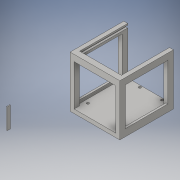
# Autodesk Inventor part: Frame_+_Slide_Top
Saved by Autodesk Inventor 2016 (Build 200138000, 138)
## iProperties
Created: 2018-09-16
Part Number: Frame_+_Slide_Top
Material: Generic
Document SubType Name: Modeling
Designer: Kyle
Density: 1 g/cm^3
Appearance: Default
Author: Kyle
Autodesk Inventor part; units mm, degrees
ref_plane "YZ Plane" through (0, 0, 0) normal (1, 0, 0) x (0, 1, 0)
ref_plane "XZ Plane" through (0, 0, 0) normal (0, 1, 0) x (-1, 0, 0)
ref_plane "XY Plane" through (0, 0, 0) normal (0, 0, 1) x (1, 0, 0)
sketch "Sketch1" plane through (0, 0, 0) normal (0, 1, 0) x (-1, 0, 0)
  line L0 (-26.5, 34) -> (26.5, 34)
  line L1 (26.5, 34) -> (26.5, -34)
  line L2 (26.5, -34) -> (-26.5, -34)
  line L3 (-26.5, -34) -> (-26.5, 34)
  line L4 (-26.5, 34) -> (26.5, -34) construction
  line L5 (26.5, 34) -> (-26.5, -34) construction
  line L6 (26.5, 34) -> (26.5, 19)
  line L7 (-26.5, -34) -> (-19.5, -34)
  line L8 (-26.5, -34) -> (8.5, -34)
  circle A0 centre (8.5, -31.5) radius 1.5
  circle A1 centre (-19.5, -31.5) radius 1.5
  line L9 (-19.5, -33) -> (-19.5, -34)
  line L10 (8.5, -33) -> (8.5, -34)
  circle A2 centre (-19.5, -31.5) radius 1.5
  circle A3 centre (24, 19) radius 1.5
  line L11 (25.5, 19) -> (26.5, 19)
  line L12 (26.5, 19) -> (25.5, 19)
  line L13 (24, 19) -> (0, 19)
  line L14 (0, 19) -> (0, 0)
  line L15 (0, 0) -> (8.5, -31.5)
  line L16 (8.5, -31.5) -> (0, -31.5)
  line L17 (-19.5, -31.5) -> (-19.5, 0)
  line L18 (-19.5, 0) -> (0, 0)
  line L19 (26.5, 34) -> (31.5, 34)
  line L20 (-31.5, -34) -> (31.5, -34)
  line L21 (31.5, -34) -> (31.5, 34)
  line L22 (31.5, 34) -> (-31.5, 34)
  line L23 (-31.5, 34) -> (-31.5, -34)
  line L24 (-31.5, -34) -> (31.5, 34) construction
  line L25 (31.5, -34) -> (-31.5, 34) construction
  dimension "d5" = 3
  dimension "d6" = 3
  dimension "d7" = 3
  dimension "d0" = 53
  dimension "d1" = 68
  dimension "d2" = 15
  dimension "d3" = 7
  dimension "d4" = 35
  dimension "d8" = 1
  dimension "d9" = 1
  dimension "d10" = 5
  constraints: 52 end point, 5 parallel, 5 perpendicular, 5 point on line, 4 midpoint, 3 horizontal, 2 vertical, 2 vertical alignment, 1 centre point, 1 coincident, 1 collinear, 1 horizontal alignment, 7 other
  measures "d0" distance of L1.end L2.end
  measures "d1" distance of L0.end L1.end
  measures "d2" distance of L0.end L6.end
  measures "d3" distance of L2.end L7.end
  measures "d4" distance of L2.end L8.end
  measures "d8" distance of L10.start L8.end
  measures "d9" distance of L11.start L6.end
  measures "d10" distance of L0.end L19.end
extrude "Extrusion1" add sketch "Sketch1" along normal blind 5 contours L0 L1 L11 A3 L13 L14 L18 L17 A1 L9 L2 L3 | L3 L20 L23 L22 | L19 L21 L20 L1 | L1 L2 L10 A0 L15 L14 L13 A3 L11 | L9 A1 L17 L18 L15 A0 L10 L2
sketch "Sketch2" plane through (0, 0, 0) normal (0, 1, 0) x (-1, 0, 0)
  line L0 (51.0115, 95.1402) -> (50.0115, 95.1402)
  line L1 (50.0115, 95.1402) -> (50.0115, 90.9953)
  line L2 (50.0115, 90.9953) -> (51.0115, 90.9953)
  line L3 (51.0115, 90.9953) -> (51.0115, 95.1402)
  point P0 (0, 0)
  dimension "d13" = 1
  constraints: 8 end point, 2 parallel, 1 horizontal, 1 perpendicular
  measures "d13" distance of L2.end L1.end
extrude "Extrusion2" add sketch "Sketch2" along normal blind 26
sketch "Sketch3" plane through (0, 5, 0) normal (0, 1, 0) x (1, 0, 0)
  line L0 (31.5, -34) -> (-31.5, -34)
  line L1 (-31.5, -34) -> (-31.5, 34)
  line L2 (-31.5, 34) -> (31.5, 34)
  line L3 (31.5, 34) -> (31.5, -34)
  line L4 (31.5, -34) -> (-31.5, 34) construction
  line L5 (-31.5, -34) -> (31.5, 34) construction
  line L6 (-31.5, -34) -> (31.5, -34) projected
  line L7 (-31.5, 34) -> (-26.5, 34)
  line L8 (-26.5, 34) -> (-26.5, -34)
  line L9 (-26.5, -34) -> (-31.5, -34)
  line L10 (-31.5, -34) -> (-31.5, 34)
  line L11 (31.5, -34) -> (31.5, 34) projected
  line L12 (31.5, 34) -> (26.5, 34)
  line L13 (26.5, 34) -> (26.5, -34)
  line L14 (26.5, -34) -> (31.5, -34)
  line L15 (31.5, -34) -> (31.5, 34)
  line L16 (-31.5, -34) -> (-26.5, -34)
  line L17 (-26.5, -34) -> (-26.5, -27)
  line L18 (-26.5, -27) -> (-31.5, -27)
  line L19 (-31.5, -27) -> (-31.5, -34)
  line L20 (-31.5, 34) -> (-26.5, 34)
  line L21 (-26.5, 34) -> (-26.5, 27)
  line L22 (-26.5, 27) -> (-31.5, 27)
  line L23 (-31.5, 27) -> (-31.5, 34)
  line L24 (31.5, 34) -> (26.5, 34)
  line L25 (26.5, 34) -> (26.5, 27)
  line L26 (26.5, 27) -> (31.5, 27)
  line L27 (31.5, 27) -> (31.5, 34)
  line L28 (26.5, -34) -> (31.5, -34)
  line L29 (31.5, -34) -> (31.5, -27)
  line L30 (31.5, -27) -> (26.5, -27)
  line L31 (26.5, -27) -> (26.5, -34)
  point P0 (0, 0)
  dimension "d16" = 5
  dimension "d17" = 5
  dimension "d18" = 5
  dimension "d19" = 7
  dimension "d20" = 5
  dimension "d21" = 7
  dimension "d22" = 5
  dimension "d23" = 7
  dimension "d24" = 5
  dimension "d25" = 7
  constraints: 60 end point, 14 parallel, 7 horizontal, 7 perpendicular, 2 midpoint, 2 point on line
  measures "d16" distance of L8.end L9.end
  measures "d17" distance of L14.end L13.end
  measures "d18" distance of L18.end L17.end
  measures "d19" distance of L17.end L16.end
  measures "d20" distance of L21.end L22.end
  measures "d21" distance of L20.end L21.end
  measures "d22" distance of L26.end L25.end
  measures "d23" distance of L25.end L24.end
  measures "d24" distance of L30.end L29.end
  measures "d25" distance of L29.end L28.end
extrude "Extrusion3" add sketch "Sketch3" along normal blind 52 contours L0 L13 L30 L3 | L0 L1 L18 L8 | L26 L13 L2 L3 | L22 L1 L2 L8
sketch "Sketch4" plane through (0, 5, 0) normal (0, 1, 0) x (1, 0, 0)
  line L0 (-31.5, 27) -> (-31.5, -27) projected
  line L1 (-26.5, -27) -> (-26.5, -34) projected
  line L2 (-31.5, 27) -> (-26.5, 27)
  line L3 (-26.5, 27) -> (-26.5, -27)
  line L4 (-26.5, -27) -> (-31.5, -27)
  line L5 (-31.5, -27) -> (-31.5, 27)
  line L6 (31.5, -27) -> (31.5, 27) projected
  line L7 (31.5, 27) -> (26.5, 27)
  line L8 (26.5, 27) -> (26.5, -27)
  line L9 (26.5, -27) -> (31.5, -27)
  line L10 (31.5, -27) -> (31.5, 27)
  line L11 (31.5, -27) -> (26.5, -27) projected
  line L12 (31.5, 27) -> (29, 27)
  line L13 (29, 27) -> (29, -27)
  line L14 (29, -27) -> (31.5, -27)
  line L15 (31.5, -27) -> (31.5, 27)
  line L16 (-26.5, -27) -> (-31.5, -27) projected
  line L17 (-31.5, 27) -> (-29, 27)
  line L18 (-29, 27) -> (-29, -27)
  line L19 (-29, -27) -> (-31.5, -27)
  line L20 (-31.5, -27) -> (-31.5, 27)
  point P0 (0, 0)
  constraints: 32 end point, 8 parallel, 4 horizontal, 4 perpendicular, 2 midpoint
extrude "Extrusion4" add sketch "Sketch4" along normal blind 4 contours L2 L18 L4 L0 | L9 L13 L7 L6
sketch "Sketch5" plane through (0, 57, 0) normal (0, 1, 0) x (1, 0, 0)
  line L0 (31.5, 34) -> (-31.5, 34) projected
  line L1 (-26.5, -34) -> (-26.5, -27) projected
  line L2 (-31.5, 34) -> (-26.5, 34)
  line L3 (-26.5, 34) -> (-26.5, -34)
  line L4 (-26.5, -34) -> (-31.5, -34)
  line L5 (-31.5, -34) -> (-31.5, 34)
  line L6 (-26.5, -27) -> (31.5, -27)
  line L7 (31.5, -27) -> (31.5, -34)
  line L8 (31.5, -34) -> (-26.5, -34)
  line L9 (-26.5, -34) -> (-26.5, -27)
  line L10 (26.5, -27) -> (26.5, -34) projected
  line L11 (26.5, -27) -> (31.5, -27)
  line L12 (31.5, -27) -> (31.5, 34)
  line L13 (31.5, 34) -> (26.5, 34)
  line L14 (26.5, 34) -> (26.5, -27)
  line L15 (-26.5, 27) -> (-26.5, 34) projected
  line L16 (-26.5, 34) -> (-26.5, 27)
  line L17 (26.5, 27) -> (26.5, 34)
  point P0 (0, 0)
  constraints: 28 end point, 7 parallel, 3 horizontal, 3 perpendicular, 1 point on line
extrude "Extrusion5" add sketch "Sketch5" along normal blind 8 contours L12 L6 L14 L0 | L7 L8 L10 L6 | L3 L1 L4 L5 L0 | L10 L8 L1 L6
sketch "Sketch6" plane through (31.5, 0, -34) normal (0, 0, -1) x (-1, 0, 0)
  line L0 (0, 0) -> (0, 65) projected
  line L1 (5, 5) -> (5, 57) projected
  line L2 (0, 65) -> (5, 65)
  line L3 (5, 63) -> (5, 60)
  line L4 (5, 57) -> (0, 57)
  line L5 (0, 57) -> (0, 65)
  line L6 (58, 5) -> (58, 57) projected
  line L7 (63, 0) -> (63, 65) projected
  line L8 (58, 57) -> (63, 57)
  line L9 (63, 57) -> (63, 65)
  line L10 (63, 65) -> (58, 65)
  line L11 (58, 65) -> (58, 57)
  line L12 (5, 57) -> (5, 60)
  line L13 (5, 5) -> (5, 65) projected
  line L14 (5, 60) -> (2.5, 60)
  line L15 (2.5, 60) -> (2.5, 63)
  line L16 (2.5, 63) -> (5, 63)
  line L17 (58, 57) -> (5, 57) projected
  line L18 (58, 57) -> (60.5, 57)
  line L19 (63, 57) -> (58, 57) projected
  line L20 (60.5, 60) -> (58, 60)
  line L21 (58, 5) -> (58, 65) projected
  line L22 (58, 60) -> (58, 63)
  line L23 (58, 63) -> (60.5, 63)
  line L24 (60.5, 63) -> (60.5, 60)
  line L25 (5, 63) -> (5, 60)
  point P0 (31.5, 0)
  point P1 (59.25, 63)
  point P2 (59.25, 60)
  dimension "d32" = 3
  dimension "d33" = 3
  constraints: 36 end point, 7 perpendicular, 4 parallel, 4 point on line, 3 midpoint, 2 horizontal, 1 collinear, 1 vertical, 2 other
  measures "d32" distance of L3.end L1.end
  measures "d33" distance of L14.end L15.end
extrude "Extrusion6" cut sketch "Sketch6" against normal up to surface (61 mm away) contours L14 L15 L16 L3 | L23 L24 L20 L11
sketch "Sketch7" plane through (26.5, 57, 27) normal (0, 0, -1) x (-1, 0, 0)
  line L0 (-2.5, 3) -> (-2.5, 6) projected
  line L1 (55.5, 3) -> (53, 3) projected
  line L2 (-2.5, 6) -> (55.5, 6)
  line L3 (55.5, 6) -> (55.5, 3)
  line L4 (55.5, 3) -> (-2.5, 3)
  line L5 (-2.5, 3) -> (-2.5, 6)
  point P0 (26.5, -57)
  constraints: 8 end point, 2 parallel, 1 horizontal, 1 perpendicular
extrude "Extrusion7" cut sketch "Sketch7" against normal blind 2.5
body "Solid1"
